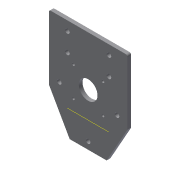
# Autodesk Inventor part: TOTEM_Base_Slide_x_20mmrod
Saved by Autodesk Inventor 2019.4 (Build 234330000, 330)
## iProperties
Created: 2021-10-12
Part Number: TOTEM_Base_Slide_x_20mmrod
Material: Generic
Document SubType Name: Modeling
Designer: diederichbenedict
Density: 1 g/cm^3
Appearance: Default
Author: diederichbenedict
Autodesk Inventor part; units mm, degrees
ref_plane "YZ Plane" through (0, 0, 0) normal (1, 0, 0) x (0, 1, 0)
ref_plane "XZ Plane" through (0, 0, 0) normal (0, 1, 0) x (-1, 0, 0)
ref_plane "XY Plane" through (0, 0, 0) normal (0, 0, 1) x (1, 0, 0)
sketch "Sketch1" plane through (0, 0, 0) normal (0, 0, 1) x (1, 0, 0)
  line L0 (0, 0) -> (-20, 0)
  line L1 (-20, 0) -> (-42.5, 40)
  line L2 (-42.5, 40) -> (-42.5, 110)
  line L3 (-42.5, 110) -> (0, 110)
  circle A0 centre (0, 8) radius 2.45
  circle A1 centre (-31.25, 48) radius 2.45
  circle A2 centre (0, 56) radius 10.1211
  line L4 (16, 72) -> (-16, 72) construction
  line L5 (-16, 72) -> (-16, 40) construction
  line L6 (-16, 40) -> (16, 40) construction
  line L7 (16, 40) -> (16, 72) construction
  line L8 (16, 72) -> (-16, 40) construction
  line L9 (-16, 72) -> (16, 40) construction
  circle A3 centre (-16, 72) radius 1.45
  circle A4 centre (-16, 40) radius 1.4
  circle A5 centre (-22.5, 100) radius 2.45
  circle A6 centre (-22.5, 80) radius 2.45
  line L10 (0, 110) -> (0, 66.1211)
  line L11 (0, 45.8789) -> (0, 10.45)
  line L12 (0, 5.55) -> (0, 0)
  dimension "d0" = 20
  dimension "d2" = 40
  dimension "d3" = 70
  dimension "d4" = 4.9
  dimension "d5" = 4.9
  dimension "d6" = 32
  dimension "d7" = 32
  dimension "d8" = 8
  dimension "d9" = 40
  dimension "d10" = 8
  dimension "d11" = 2.9
  dimension "d12" = 2.8
  dimension "d13" = 4.9
  dimension "d14" = 4.9
  dimension "d15" = 10
  dimension "d16" = 30
  dimension "d17" = 20
  dimension "d18" = 20
  constraints: 26 end point, 7 centre point, 6 perpendicular, 4 point on circle, 2 coincident, 2 horizontal, 2 midpoint, 2 parallel
  measures "d0" distance of L0.start L0.end
  measures "d2" vertical distance of L0.end L1.end
  measures "d3" distance from line of L1.end L3
  measures "d4" diameter of A0
  measures "d5" diameter of A1
  measures "d6" distance of L6.end L5.end
  measures "d7" distance of L5.end L4.end
  measures "d8" distance from line of L0 A0.centre
  measures "d9" vertical distance of A1.centre A0.centre
  measures "d10" vertical distance of A2.centre A1.centre
  measures "d11" diameter of A3
  measures "d12" diameter of A4
  measures "d13" diameter of A5
  measures "d14" diameter of A6
  measures "d15" distance from line of A5.centre L3
  measures "d16" distance from line of L3 A6.centre
  measures "d17" distance from line of A5.centre L2
  measures "d18" distance from line of L2 A6.centre
extrude "Extrusion1" add sketch "Sketch1" along normal blind 4 contours L0 L1 L2 L3 L10 A2 L11 A0 L12
fillet "Fillet1" radius 2 1 edges at (-42.5, 110, 2)
mirror "Mirror1" about plane through (0, 66.1211, 0) normal (1, 0, 0) of "Extrusion1", "Fillet1"
ref_plane "Work Plane1" through (-20, 28, 0) normal (0, -1, 0) x (1, 0, 0)
equation "\"d17\" = d18"
body "Solid1"
